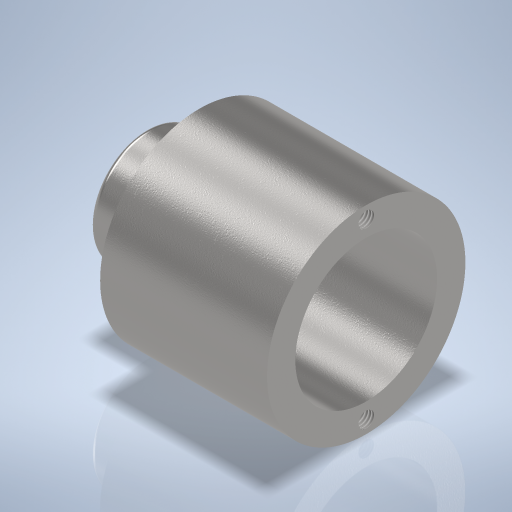
# Autodesk Inventor part: Zylinder
Saved by Autodesk Inventor 2024 (Build 280153000, 153)
## iProperties
Created: 2024-02-29
Part Number: Zylinder
Material: Stahl, galvanisiert
Document SubType Name: Modeling
Designer: ffogue
Density: 7.85 g/cm^3
Appearance: Galvanisiert
Author: ffogue
Autodesk Inventor part; units mm, degrees
note: some values were not read from the file. Chosen so that the rebuilt part matches the saved one: direction of "Bohrung5".
ref_plane "YZ Plane" through (0, 0, 0) normal (1, 0, 0) x (0, 1, 0)
ref_plane "XZ Plane" through (0, 0, 0) normal (0, 1, 0) x (-1, 0, 0)
ref_plane "XY Plane" through (0, 0, 0) normal (0, 0, 1) x (1, 0, 0)
sketch "Skizze1" plane through (0, 0, 0) normal (0, 0, 1) x (1, 0, 0)
  line L0 (0, 0) -> (0, 18)
  line L1 (0, 18) -> (17, 18)
  line L2 (17, 18) -> (17, 31.5)
  line L3 (17, 31.5) -> (70, 31.5)
  line L4 (70, 31.5) -> (70, 0)
  line L5 (70, 0) -> (0, 0)
  dimension "d0" = 70
  dimension "d1" = 36
  dimension "d2" = 17
  dimension "d3" = 63
  constraints: 12 end point, 5 perpendicular, 1 vertical
  measures "d0" distance between parallel lines of L4 L0
  measures "d1" diameter of L1 L5
  measures "d2" distance between parallel lines of L2 L0
  measures "d3" diameter of L3 L5
revolve "Umdrehung1" add sketch "Skizze1" angle 360 about axis through (70, 0, 0) along (-1, 0, 0)
sketch "Skizze2" plane through (70, 0, 0) normal (1, 0, 0) x (0, 0, -1)
  circle A0 centre (0, 0) radius 22.5
  dimension "d5" = 45
  constraints: 1 centre point, 1 coincident
  measures "d5" diameter of A0
extrude "Extrusion1" cut sketch "Skizze2" against normal blind 40
sketch "Skizze8" plane through (70, 0, 0) normal (1, 0, 0) x (0, 0, -1)
  line L0 (0, 0) -> (0, 31.8712) construction
  point P0 (-27.5, 0)
  point P1 (27.5, 0)
  dimension "d38" = 55
  constraints: 2 end point, 1 horizontal alignment, 1 symmetric about line, 1 vertical
  measures "d38" distance of point (27.5, 0) point (-27.5, 0)
hole "Bohrung5" at (70, 0, 27.5) at (70, 0, -27.5) direction (-1, 0, 0) diameter 4.917 depth 53 thread size "M6x1" class "6H" standard "ISO Metric profile"
fillet "Rundung1" radius 2 1 edges at (0, -18, 0)
sketch "Skizze3" plane through (30, 0, 0) normal (1, 0, 0) x (0, 0, -1)
  line L0 (0, 0) -> (0, 13.1561) construction
  point P0 (-10, 0)
  point P1 (10, 0)
  dimension "d8" = 20
  constraints: 2 end point, 1 horizontal alignment, 1 symmetric about line, 1 vertical
  measures "d8" distance of point (10, 0) point (-10, 0)
sketch "Skizze4" plane through (30, 0, 0) normal (1, 0, 0) x (0, 0, -1)
  circle A0 centre (10, 0) radius 2 projected
  point P0 (0, 0)
  point P1 (10, 0)
  constraints: 1 coincident
sketch "Skizze6" plane through (0, 0, 0) normal (-1, 0, 0) x (0, 0, 1)
  circle A0 centre (10, 0) radius 2 projected
  point P0 (0, 0)
  point P1 (10, 0)
  constraints: 1 coincident
sketch "Skizze5" plane through (0, 0, 0) normal (-1, 0, 0) x (0, 0, 1)
  circle A0 centre (-10, 0) radius 2 projected
  point P0 (0, 0)
  point P1 (-10, 0)
  constraints: 1 coincident
